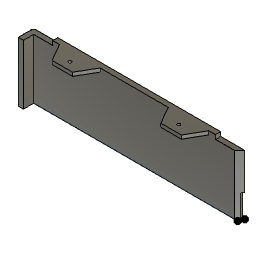
Front Wall v7 (Autodesk Fusion 360 design; units mm, degrees)
Autodesk Fusion 360 part; units mm, degrees
note: some values were not read from the file. Set by a fixed rule: which sketch regions a step uses.
sketch "Sketch1" plane through (0, 0, 0) normal (0, 0, 1) x (1, 0, 0)
  line L0 (-156.1, 40) -> (50, 40)
  line L1 (50, 40) -> (50, 35)
  line L2 (50, 35) -> (-156.1, 35)
  line L3 (-156.1, 35) -> (-156.1, 40)
  circle A0 centre (-106.1, 25.5) radius 1.5
  circle A1 centre (0, 25.5) radius 1.5
  line L4 (-116.1, 35) -> (-96.1, 35)
  line L5 (-96.1, 35) -> (-96.1, 18)
  line L6 (-96.1, 18) -> (-116.1, 18)
  line L7 (-116.1, 18) -> (-116.1, 35)
  line L8 (-10, 35) -> (10, 35)
  line L9 (10, 35) -> (10, 18)
  line L10 (10, 18) -> (-10, 18)
  line L11 (-10, 18) -> (-10, 35)
  line L12 (-96.1, 18) -> (-86.285, 35)
  line L13 (-116.1, 18) -> (-125.915, 35)
  line L14 (-10, 18) -> (-19.815, 35)
  line L15 (10, 18) -> (19.815, 35)
  line L16 (50, 40) -> (45, 35)
  dimension "d1" = 206.1
  dimension "d2" = 5
  dimension "d3" = 3
  dimension "d4" = 3
  dimension "d5" = 50
  dimension "d6" = 14.5
  dimension "d7" = 50
  dimension "d8" = 14.5
  dimension "d9" = 10
  dimension "d10" = 10
  dimension "d11" = 7.5
  dimension "d12" = 10
  dimension "d13" = 10
  dimension "d14" = 7.5
  dimension "d15" = 30
  dimension "d16" = 30
  dimension "d17" = 30
  dimension "d18" = 30
  dimension "d19" = 45
  constraint horizontal L0
  constraint vertical L1
  constraint horizontal L2
  constraint vertical L3
  constraint horizontal L4
  constraint vertical L5
  constraint horizontal L6
  constraint vertical L7
  constraint coincident L2 L4.start
  constraint horizontal L8
  constraint vertical L9
  constraint horizontal L10
  constraint vertical L11
  constraint coincident L2 L8.start
  constraint coincident L2 L12.end
  constraint coincident L2 L13.end
  constraint coincident L2 L14.end
  constraint coincident L2 L15.end
  constraint coincident L2 L16.end
  measures "d1" distance of L1 L3
  measures "d2" distance of L0.start L2.end
  measures "d3" diameter of A0
  measures "d4" diameter of A1
  measures "d5" distance of L3 A0.centre
  measures "d6" distance of L0 A0.centre
  measures "d7" distance of L1 A1.centre
  measures "d8" distance of L0 A1.centre
  measures "d9" distance of A1.centre L11
  measures "d10" distance of A1.centre L9
  measures "d11" distance of A1.centre L10
  measures "d12" distance of A0.centre L5
  measures "d13" distance of A0.centre L7
  measures "d14" distance of A0.centre L6
  measures "d15" angle of L7 L13
  measures "d16" angle of L5 L12
  measures "d17" angle of L11 L14
  measures "d18" angle of L9 L15
  measures "d19" angle of L1 L16
extrude "Extrude1" add sketch "Sketch1" against normal blind 3.5 contours L2 L7 L13 | L2 L9 L15 | L2 L4 L5 L6 L7 | L2 L8 L9 L10 L11 | L2 L5 L12 | L2 L11 L14 makes body 1 at (-95.6839, 26.314, 0) makes body 2 at (10.4161, 26.314, 0)
extrude "Extrude2" add sketch "Sketch1" against normal blind 62.2 contours L0 L2 L3 L4 L8 L16 bodies 1 2
sketch "Sketch3" plane through (0, 0, 0) normal (0, 0, 1) x (-1, 0, 0)
  circle A0 centre (0, -25.5) radius 1.5
  circle A1 centre (106.1, -25.5) radius 1.5
  line L0 (96.1, -18) -> (86.285, -35)
  line L1 (86.285, -35) -> (19.815, -35)
  line L2 (19.815, -35) -> (10, -18)
  line L3 (10, -18) -> (-10, -18)
  line L4 (-10, -18) -> (-19.815, -35)
  line L5 (-19.815, -35) -> (-45, -35)
  line L6 (-45, -35) -> (-50, -40)
  line L7 (-50, -40) -> (156.1, -40)
  line L8 (125.915, -35) -> (116.1, -18)
  line L9 (116.1, -18) -> (96.1, -18)
  line L10 (-50, -40) -> (-26.5, -40)
  line L11 (-26.5, -40) -> (-26.5, -35)
  line L12 (-26.5, -35) -> (-50, -35)
  line L13 (-50, -35) -> (-50, -40)
  line L14 (156.1, -40) -> (132.6, -40)
  line L15 (132.6, -40) -> (132.6, -35)
  line L16 (132.6, -35) -> (156.1, -35)
  line L17 (156.1, -35) -> (156.1, -40)
  line L18 (156.1, -40) -> (156.1, -35)
  line L19 (156.1, -35) -> (125.915, -35)
  dimension "d28" = 5
  dimension "d29" = 23.5
  dimension "d30" = 5
  dimension "d31" = 23.5
  constraint horizontal L10
  constraint vertical L11
  constraint horizontal L12
  constraint vertical L13
  constraint coincident L5 L11.end
  constraint coincident L6.end L7.start
  constraint horizontal L14
  constraint vertical L15
  constraint horizontal L16
  constraint vertical L17
  constraint coincident L7.end L14.start
  measures "d28" distance of L7.end L16.end
  measures "d29" distance of L15 L17
  measures "d30" distance of L10 L12
  measures "d31" distance of L11 L13
extrude "Extrude3" cut sketch "Sketch3" against normal blind 4 contours L7 L14 L15 L16 L17 L18 L19 | L5 L6 L7 L10 L11 L12 bodies 1
sketch "Sketch4" plane through (0, 0, -62.2) normal (0, 0, -1) x (1, 0, 0)
  line L0 (45, -35) -> (-156.1, -35)
  line L1 (-156.1, -35) -> (-156.1, -40)
  line L2 (-156.1, -40) -> (50, -40)
  line L3 (50, -40) -> (45, -35)
  line L4 (50, -40) -> (48, -40)
  line L5 (48, -40) -> (48, -35)
  line L6 (48, -35) -> (50, -35)
  line L7 (50, -35) -> (50, -40)
  dimension "d34" = 5
  dimension "d35" = 2
  constraint horizontal L4
  constraint vertical L5
  constraint horizontal L6
  constraint vertical L7
  constraint coincident L0 L5.end
  constraint coincident L2.end L3.start
  measures "d34" distance of L4 L6
  measures "d35" distance of L5 L7
extrude "Extrude5" cut sketch "Sketch4" against normal blind 22.4 contours L2 L3 L4 L5 bodies 1
sketch "Sketch5" plane through (0, 35, 0) normal (0, -1, 0) x (1, 0, 0)
  line L0 (-132.6, -4) -> (-156.1, -4)
  line L1 (-156.1, -4) -> (-156.1, -62.2)
  line L2 (-156.1, -62.2) -> (45, -62.2)
  line L3 (45, -62.2) -> (45, -4)
  line L4 (45, -4) -> (26.5, -4)
  line L5 (26.5, -4) -> (26.5, 0)
  line L6 (26.5, 0) -> (19.815, 0)
  line L7 (19.815, 0) -> (19.815, -3.5)
  line L8 (19.815, -3.5) -> (-19.815, -3.5)
  line L9 (-19.815, -3.5) -> (-19.815, 0)
  line L10 (-19.815, 0) -> (-86.285, 0)
  line L11 (-86.285, 0) -> (-86.285, -3.5)
  line L12 (-86.285, -3.5) -> (-125.915, -3.5)
  line L13 (-125.915, -3.5) -> (-125.915, 0)
  line L14 (-125.915, 0) -> (-132.6, 0)
  line L15 (-132.6, 0) -> (-132.6, -4)
  line L16 (-156.1, -4) -> (-151.1, -4)
  line L17 (-151.1, -4) -> (-151.1, -62.2)
  line L18 (-151.1, -62.2) -> (-156.1, -62.2)
  line L19 (-156.1, -62.2) -> (-156.1, -4)
  dimension "d40" = 5
  constraint horizontal L16
  constraint vertical L17
  constraint horizontal L18
  constraint vertical L19
  constraint coincident L2 L17.end
  constraint coincident L0.end L1.start
  measures "d40" distance of L17 L19
extrude "Extrude6" add sketch "Sketch5" along normal blind 10 contours L0 L1 L2 L16 L17 L18 L19 bodies 1
fillet "Fillet1" radius 2 1 edges at (-156.1, 40, -33.1) on bodies 1
